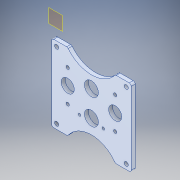
# Autodesk Inventor part: am-2725+3CIM4U+Motor+Plate+r2
Saved by Autodesk Inventor 2018 (Build 220112000, 112)
## iProperties
Created: 2014-01-23
Part Number: am-2725+3CIM4U+Motor+Plate+r2
Material: Generic
Description: STEP AP214
Document SubType Name: Modeling
Designer: S-2512711
Density: 1 g/cm^3
Appearance: Default
Sending System: SolidWorks 2010
Preprocessor: SwSTEP 2.0
Title: am-2725 3CIM4U Motor Plate r2.STEP
Revision Number: ANY
Autodesk Inventor part; units mm, degrees
ref_plane "YZ Plane" through (0, 0, 0) normal (1, 0, 0) x (0, 1, 0)
ref_plane "XZ Plane" through (0, 0, 0) normal (0, 1, 0) x (-1, 0, 0)
ref_plane "XY Plane" through (0, 0, 0) normal (0, 0, 1) x (1, 0, 0)
ref_plane "Work Plane1" through (-63.5, 101.6, 34.925) normal (0, 0, 1) x (1, 0, 0)
sketch "Sketch2" plane through (-63.5, 101.6, 34.925) normal (0, 0, 1) x (1, 0, 0)
  circle A0 centre (63.5, -101.6) radius 11.1125
  circle A1 centre (44.45, -106.3625) radius 2.0193 projected
  circle A2 centre (44.45, -106.3625) radius 2.0193
  circle A3 centre (25.5848, -101.08) radius 2.54 projected
  circle A4 centre (25.5848, -101.08) radius 2.54
  line L0 (44.45, -106.3625) -> (82.55, -106.3625)
  circle A5 centre (82.55, -106.3625) radius 2.0193
  circle A6 centre (101.4152, -101.08) radius 2.54 projected
  line L1 (25.5848, -101.08) -> (101.4152, -101.08)
  circle A7 centre (101.4152, -101.08) radius 2.54
  line L2 (25.5848, -101.08) -> (25.5848, -75.68)
  line L3 (101.4152, -101.08) -> (101.4152, -75.68)
  circle A8 centre (25.5848, -75.68) radius 10.414
  circle A9 centre (101.4152, -75.68) radius 10.414
  circle A10 centre (63.5, -60.9092) radius 11.1125 projected
  line L4 (63.5, -60.9092) -> (63.5, -101.6)
  circle A11 centre (63.5, -60.9092) radius 11.1125
  circle A12 centre (25.5848, -50.28) radius 2.54 projected
  line L5 (25.5848, -50.28) -> (25.5848, -75.68)
  line L6 (101.4152, -75.68) -> (101.4152, -50.28)
  circle A13 centre (25.5848, -50.28) radius 2.54
  circle A14 centre (101.4152, -50.28) radius 2.54
  circle A15 centre (63.5, -101.6) radius 11.1125 projected
  line L7 (127, 0) -> (127, -139.7) projected
  line L8 (0, -139.7) -> (0, 0) projected
  line L9 (0, -144.9324) -> (127, -144.9324)
  line L10 (0, -144.9324) -> (7.9248, -144.9324)
  line L11 (7.9248, -144.9324) -> (7.9248, -137.0076)
  circle A16 centre (7.9248, -137.0076) radius 3.2512
  line L12 (127, -144.9324) -> (119.0752, -144.9324)
  line L13 (119.0752, -144.9324) -> (119.0752, -137.0076)
  circle A17 centre (119.0752, -137.0076) radius 3.2512
  line L14 (0, 0) -> (127, 0) projected
  line L15 (0, -22.6568) -> (127, -22.6568)
  line L16 (0, -22.6568) -> (7.9248, -22.6568)
  line L17 (7.9248, -22.6568) -> (7.9248, -30.5816)
  line L18 (127, -22.6568) -> (119.0752, -22.6568)
  line L19 (119.0752, -22.6568) -> (119.0752, -30.5816)
  circle A18 centre (7.9248, -30.5816) radius 3.2512
  circle A19 centre (119.0752, -30.5816) radius 3.2512
  line L20 (63.5, 0) -> (63.5, -17.78)
  line L21 (0, -144.9324) -> (0, -22.6568)
  line L22 (127, -144.9324) -> (127, -22.6568)
  line L23 (63.5, -101.6) -> (63.5, -106.3625)
  line L24 (63.5, -106.3625) -> (82.55, -106.3625)
  line L25 (82.55, -106.3625) -> (44.45, -106.3625)
  dimension "d0" = 38.1
  dimension "d1" = 25.4
  dimension "d23" = 7.9248
  dimension "d24" = 7.9248
  dimension "d25" = 17.78
  dimension "d27" = 38.2524
  dimension "d29" = 7.9248
  dimension "d30" = 7.9248
  dimension "d31" = 43.3324
  constraints: 46 end point, 14 centre point, 14 coincident, 8 point on line, 7 vertical, 5 perpendicular, 3 collinear, 3 concentric, 2 horizontal, 2 midpoint
  measures "d0" distance of L0.start L0.end
  measures "d1" distance of L1.start L2.end
  measures "d23" distance of L10.end L11.end
  measures "d24" distance of L12.end L13.end
  measures "d25" distance of L20.start L20.end
  measures "d27" distance from line of L15 A11.centre
  measures "d29" distance of L16.end L17.end
  measures "d30" distance of L18.end L19.end
  measures "d31" distance from line of L9 point (63.5, -101.6)
extrude "Extrusion1" add sketch "Sketch2" along normal blind 6.35 contours L7 L22 L9 L21 L8 L15
fillet "Fillet1" radius 3.175 4 edges at (-63.5, 78.9432, 38.1) (-63.5, -43.3324, 38.1) (63.5, 78.9432, 38.1) (63.5, -43.3324, 38.1)
sketch "Sketch5" plane through (-63.5, 101.6, 41.275) normal (0, 0, 1) x (1, 0, 0)
  line L0 (3.175, -144.9324) -> (123.825, -144.9324) projected
  line L1 (63.5, -144.9324) -> (25.4, -144.9324)
  line L2 (25.4, -144.9324) -> (101.6, -144.9324)
  line L3 (63.5, -144.9324) -> (63.5, -124.6124)
  arc A0 (101.6, -144.9324) -> (25.4, -144.9324) centre (63.5, -170.4912) ccw
  line L4 (123.825, -22.6568) -> (3.175, -22.6568) projected
  line L5 (25.4, -22.6568) -> (101.6, -22.6568)
  line L6 (63.5, -22.6568) -> (63.5, -41.7068)
  arc A1 (25.4, -22.6568) -> (101.6, -22.6568) centre (63.5, 5.9182) ccw
  line L7 (25.4, -144.9324) -> (101.6, -144.9324)
  arc A2 (101.6, -144.9324) -> (25.4, -144.9324) centre (63.5, -170.4912) ccw
  point P0 (63.5, -101.6)
  dimension "d16" = 38.1
  dimension "d17" = 76.2
  dimension "d18" = 20.32
  dimension "d19" = 19.05
  constraints: 12 end point, 9 point on circle, 4 point on line, 3 centre point, 2 midpoint, 2 vertical
  measures "d16" distance of L1.start L1.end
  measures "d17" distance of L1.end L2.end
  measures "d18" distance of L1.start L3.end
  measures "d19" distance of L6.start L6.end
extrude "Extrusion2" cut sketch "Sketch5" against normal blind 25.4
fillet "Fillet2" radius 3.175 4 edges at (-38.1, 78.9432, 38.1) (38.1, 78.9432, 38.1) (38.1, -43.3324, 38.1) (-38.1, -43.3324, 38.1)
body "Solid2"
